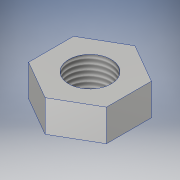
# Autodesk Inventor part: nut for baring
Saved by Autodesk Inventor 2018 (Build 220112000, 112)
## iProperties
Created: 2018-03-08
Part Number: nut for baring
Material: Aluminum 6061
Document SubType Name: Modeling
Designer: 238438
Density: 2.7 g/cm^3
Appearance: Aluminum - Flat
Mass: 0.236978 g
Surface Area: 1.64591 cm^2
Volume: 0.0877696 cm^3
Author: 238438
Autodesk Inventor part; units mm, degrees
ref_plane "YZ Plane" through (0, 0, 0) normal (1, 0, 0) x (0, 1, 0)
ref_plane "XZ Plane" through (0, 0, 0) normal (0, 1, 0) x (-1, 0, 0)
ref_plane "XY Plane" through (0, 0, 0) normal (0, 0, 1) x (1, 0, 0)
sketch "Sketch1" plane through (0, 0, 0) normal (0, 1, 0) x (-1, 0, 0)
  line L0 (0, 4.0328) -> (3.4925, 2.0164)
  line L1 (3.4925, 2.0164) -> (3.4925, -2.0164)
  line L2 (3.4925, -2.0164) -> (0, -4.0328)
  line L3 (0, -4.0328) -> (-3.4925, -2.0164)
  line L4 (-3.4925, -2.0164) -> (-3.4925, 2.0164)
  line L5 (-3.4925, 2.0164) -> (0, 4.0328)
  circle A0 centre (0, 0) radius 1.905
  dimension "d0" = 6.985
  dimension "d1" = 3.81
  constraints: 12 end point, 2 coincident, 1 centre point, 13 other
  measures "d0" distance between parallel lines of L3 L0
  measures "d1" diameter of A0
extrude "Extrusion1" add sketch "Sketch1" along normal blind 2.8448
thread "Thread1" size "2-56 UNC" class "2B" standard "ANSI Unified Screw Threads" full length
body "Solid1"
